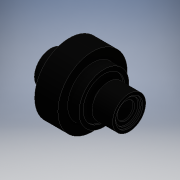
# Autodesk Inventor part: ET23
Saved by Autodesk Inventor 2016 (Build 200138000, 138)
## iProperties
Created: 2016-04-16
Part Number: ET23
Material: Genérico
Document SubType Name: Modeling
Designer: Usuario1
Density: 1 g/cm^3
Appearance: Valor por defecto
Author: Usuario1
Autodesk Inventor part; units mm, degrees
ref_plane "YZ Plane" through (0, 0, 0) normal (1, 0, 0) x (0, 1, 0)
ref_plane "XZ Plane" through (0, 0, 0) normal (0, 1, 0) x (-1, 0, 0)
ref_plane "XY Plane" through (0, 0, 0) normal (0, 0, 1) x (1, 0, 0)
sketch "Boceto1" plane through (0, 0, 0) normal (0, 0, 1) x (1, 0, 0)
  line L0 (0.448, 0) -> (0.448, -0.4011)
  line L1 (0.448, -0.4011) -> (0, -0.4011)
  line L2 (0, -0.4011) -> (0, 0)
  line L3 (1.0145, -0.8419) -> (0.448, -0.8419)
  line L4 (1.0145, -0.6065) -> (1.2916, -0.6065)
  line L5 (1.2516, 0) -> (1.2516, -0.5065)
  line L6 (1.2916, -0.6065) -> (1.2916, -0.5065)
  line L7 (1.2916, -0.5065) -> (1.2516, -0.5065)
  line L8 (1.2516, -0.2065) -> (1.4016, -0.2065)
  line L9 (1.4016, -0.2065) -> (1.4016, 0)
  line L10 (1.4016, -0.0065) -> (1.4016, -0.4011)
  line L11 (1.4016, -0.4011) -> (1.9016, -0.4011)
  line L12 (1.4016, 0) -> (1.4016, -0.2038)
  line L13 (1.9016, -0.33) -> (1.8616, -0.33)
  line L14 (1.8616, -0.29) -> (1.8216, -0.29)
  line L15 (1.8616, -0.29) -> (1.8616, -0.33)
  line L16 (1.9016, -0.33) -> (1.9016, -0.4011)
  line L17 (1.8216, -0.21) -> (1.7816, -0.21)
  arc A0 (1.7816, -0.21) -> (1.8216, 0) centre (1.2504, 0) ccw
  line L18 (1.8216, -0.21) -> (1.8216, -0.29)
  line L19 (0, 0) -> (1.8216, 0)
  line L20 (1.0145, 0) -> (1.0145, -0.7419)
  line L21 (1.0145, 0) -> (1.0145, -0.8419)
  line L22 (0.448, -0.8419) -> (0.448, 0)
  constraints: 46 end point, 13 point on line, 2 point on circle, 1 centre point, 1 midpoint
revolve "Revolución1" add sketch "Boceto1" angle 360 about axis through (0, 0, 0) along (1, 0, 0)
sketch "Boceto2" plane through (0, 0, 0) normal (-1, 0, 0) x (0, 0, 1)
  circle A0 centre (0, 0) radius 0.4011 projected
  line L0 (0, 0.17) -> (0.17, 0.17)
  line L1 (0.17, 0.17) -> (0.17, -0.17)
  line L2 (0.17, -0.17) -> (0, -0.17)
  line L3 (0, 0.17) -> (-0.17, 0.17)
  line L4 (-0.17, 0.17) -> (-0.17, -0.17)
  line L5 (-0.17, -0.17) -> (0, -0.17)
  line L6 (-0.17, -0.17) -> (0.17, -0.17)
  line L7 (0.17, -0.17) -> (0.17, 0.17)
  line L8 (0.17, 0.17) -> (-0.17, 0.17)
  line L9 (-0.17, 0.17) -> (-0.17, -0.17)
  constraints: 20 end point, 2 parallel, 2 perpendicular, 1 horizontal
extrude "Extrusión1" cut sketch "Boceto2" against normal blind 0.5 contours L0 L1 L2 L5 L4 L3
